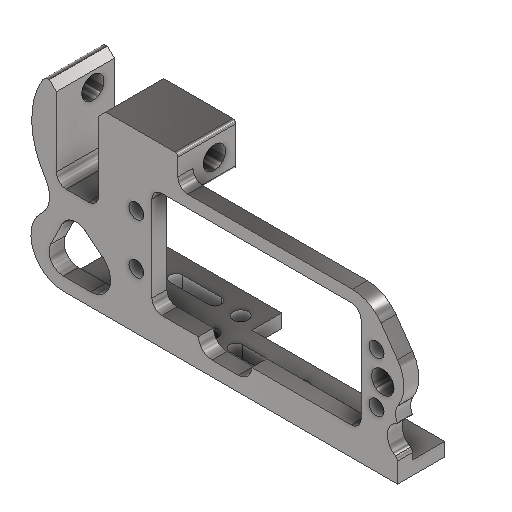
# Autodesk Inventor part: 650 서보모터 마운트
Saved by Autodesk Inventor 2026.2 (Build 302298010, 298A)
## iProperties
Created: 2026-03-24
Part Number: 650 서보모터 마운트
Material: 일반
Document SubType Name: Modeling
Designer: jh002
Density: 1 g/cm^3
Appearance: 기본값
Author: jh002
Autodesk Inventor part; units mm, degrees
ref_plane "YZ Plane" through (0, 0, 0) normal (1, 0, 0) x (0, 1, 0)
ref_plane "XZ Plane" through (0, 0, 0) normal (0, 1, 0) x (-1, 0, 0)
ref_plane "XY Plane" through (0, 0, 0) normal (0, 0, 1) x (1, 0, 0)
sketch "스케치1" plane through (0, 0, 0) normal (0, 1, 0) x (-1, 0, 0)
  line L0 (33.1, -7.725) -> (-33.1, -7.725)
  line L1 (-33.1, -7.725) -> (-33.1, 7.725)
  line L2 (-33.1, 7.725) -> (33.1, 7.725)
  line L3 (33.1, 7.725) -> (33.1, -7.725)
  line L4 (33.1, -7.725) -> (-33.1, 7.725) construction
  line L5 (-33.1, -7.725) -> (33.1, 7.725) construction
  line L6 (33.1, -1.675) -> (-33.1, -1.675)
  line L7 (5.4, -1.675) -> (5.4, -7.725)
  point P0 (0, 0)
  dimension "d0" = 66.2
  dimension "d1" = 15.45
  dimension "d2" = 9.4
  dimension "d3" = 38.5
  constraints: 16 end point, 4 point on line, 3 perpendicular, 2 midpoint, 2 parallel, 1 horizontal
  measures "d0" distance of L1.end L2.end
  measures "d1" distance of L0.end L1.end
  measures "d2" distance between parallel lines of L2 L6
  measures "d3" distance between parallel lines of L1 L7
extrude "돌출1" add sketch "스케치1" along normal blind 2.7 contours L0 L7 L6 L3 | L6 L1 L2 L3
sketch "스케치2" plane through (0, 0, 0) normal (0, -1, 0) x (1, 0, 0)
  line L0 (33.1, 7.725) -> (33.1, -1.675) projected
  line L1 (-33.1, 7.725) -> (33.1, 7.725) projected
  line L2 (-33.1, -7.725) -> (-33.1, 7.725) projected
  line L3 (-5.4, -7.725) -> (-33.1, -7.725) projected
  line L4 (-5.4, -1.675) -> (-5.4, -7.725) projected
  line L5 (33.1, -1.675) -> (-5.4, -1.675) projected
  circle A0 centre (27, 3.025) radius 1.5
  circle A1 centre (9, 3.025) radius 1.5
  circle A2 centre (-9, 3.025) radius 1.5
  line L6 (9, 3.025) -> (27, 3.025) construction
  line L7 (12.885, 3.025) -> (23.115, 3.025) construction
  line L8 (14.135, 4.275) -> (21.865, 4.275)
  line L9 (23.115, 3.025) -> (23.115, 3.025)
  line L10 (21.865, 1.775) -> (14.135, 1.775)
  line L11 (12.885, 3.025) -> (12.885, 3.025)
  line L12 (12.885, 4.275) -> (23.115, 1.775) construction
  line L13 (23.115, 4.275) -> (12.885, 1.775) construction
  arc A3 (14.135, 4.275) -> (12.885, 3.025) centre (14.135, 3.025) ccw
  arc A4 (12.885, 3.025) -> (14.135, 1.775) centre (14.135, 3.025) ccw
  arc A5 (21.865, 1.775) -> (23.115, 3.025) centre (21.865, 3.025) ccw
  arc A6 (23.115, 3.025) -> (21.865, 4.275) centre (21.865, 3.025) ccw
  line L14 (-9, 3.025) -> (9, 3.025) construction
  line L15 (-5.115, 3.025) -> (5.115, 3.025) construction
  line L16 (-3.865, 4.275) -> (3.865, 4.275)
  line L17 (5.115, 3.025) -> (5.115, 3.025)
  line L18 (3.865, 1.775) -> (-3.865, 1.775)
  line L19 (-5.115, 3.025) -> (-5.115, 3.025)
  line L20 (-5.115, 4.275) -> (5.115, 1.775) construction
  line L21 (5.115, 4.275) -> (-5.115, 1.775) construction
  arc A7 (-3.865, 4.275) -> (-5.115, 3.025) centre (-3.865, 3.025) ccw
  arc A8 (-5.115, 3.025) -> (-3.865, 1.775) centre (-3.865, 3.025) ccw
  arc A9 (3.865, 1.775) -> (5.115, 3.025) centre (3.865, 3.025) ccw
  arc A10 (5.115, 3.025) -> (3.865, 4.275) centre (3.865, 3.025) ccw
  line L22 (-23.115, 3.025) -> (-12.885, 3.025) construction
  line L23 (-21.865, 4.275) -> (-14.135, 4.275)
  line L24 (-14.135, 1.775) -> (-21.865, 1.775)
  line L25 (-23.115, 4.275) -> (-12.885, 1.775) construction
  line L26 (-12.885, 4.275) -> (-23.115, 1.775) construction
  arc A11 (-21.865, 4.275) -> (-23.115, 3.025) centre (-21.865, 3.025) ccw
  arc A12 (-23.115, 3.025) -> (-21.865, 1.775) centre (-21.865, 3.025) ccw
  arc A13 (-14.135, 1.775) -> (-12.885, 3.025) centre (-14.135, 3.025) ccw
  arc A14 (-12.885, 3.025) -> (-14.135, 4.275) centre (-14.135, 3.025) ccw
  line L27 (-9, 3.025) -> (-18, 3.025) construction
  circle A15 centre (-27, 3.025) radius 1.5
  line L28 (-7.8456, 0) -> (-28.9088, 0)
  circle A16 centre (-9, -3.025) radius 1.5
  arc A17 (-23.115, -3.025) -> (-21.865, -4.275) centre (-21.865, -3.025) ccw
  arc A18 (-21.865, -1.775) -> (-23.115, -3.025) centre (-21.865, -3.025) ccw
  line L29 (-21.865, -4.275) -> (-14.135, -4.275)
  line L30 (-14.135, -1.775) -> (-21.865, -1.775)
  line L31 (-23.115, -4.275) -> (-12.885, -1.775) construction
  line L32 (-12.885, -4.275) -> (-23.115, -1.775) construction
  arc A19 (-14.135, -4.275) -> (-12.885, -3.025) centre (-14.135, -3.025) ccw
  arc A20 (-12.885, -3.025) -> (-14.135, -1.775) centre (-14.135, -3.025) ccw
  line L33 (-23.115, -3.025) -> (-12.885, -3.025) construction
  line L34 (-9, -3.025) -> (-18, -3.025) construction
  circle A21 centre (-27, -3.025) radius 1.5
  point P0 (0, 0)
  point P1 (33.1, 3.025)
  point P2 (18, 3.025)
  point P3 (0, 3.025)
  point P4 (12.885, 3.025)
  point P5 (-5.115, 3.025)
  point P6 (-12.885, -3.025)
  point P7 (-12.885, 3.025)
  dimension "d6" = 3
  dimension "d7" = 6.1
  dimension "d8" = 3
  dimension "d9" = 18
  dimension "d10" = 3
  dimension "d11" = 18
  dimension "d24" = 10.23
  dimension "d25" = 1.25
  dimension "d26" = 10.23
  dimension "d27" = 1.25
  dimension "d135" = 10.23
  dimension "d136" = 1.25
  dimension "d137" = 9
  dimension "d138" = 3
  dimension "d139" = 18
  constraints: 58 end point, 32 point on circle, 27 point on line, 22 centre point, 21 symmetric about line, 20 tangent, 12 midpoint, 9 equal radius, 8 horizontal, 5 parallel, 2 perpendicular, 20 other
  measures "d6" diameter of A0
  measures "d7" distance of L6.end point (33.1, 3.025)
  measures "d8" diameter of A1
  measures "d9" distance of L6.end L6.start
  measures "d10" diameter of A2
  measures "d11" distance of L6.start L14.start
  measures "d24" distance of L7.start L7.end
  measures "d25" radius of A3
  measures "d26" distance of L15.start L15.end
  measures "d27" radius of A7
  measures "d135" distance of L22.start L22.end
  measures "d136" radius of A11
  measures "d137" distance of L14.start L27.end
  measures "d138" diameter of A15
  measures "d139" distance of A15.centre L14.start
sketch "스케치3" plane through (0, 2.7, 0) normal (0, 1, 0) x (1, 0, 0)
  line L0 (33.1, -7.725) -> (33.1, 1.675) projected
  line L1 (33.1, 1.675) -> (-5.4, 1.675) projected
  line L2 (-5.4, 1.675) -> (-5.4, 7.725) projected
  line L3 (-5.4, 7.725) -> (-33.1, 7.725) projected
  line L4 (-33.1, 7.725) -> (-33.1, -7.725) projected
  line L5 (-33.1, -7.725) -> (33.1, -7.725) projected
  line L6 (33.1, -4.725) -> (-33.1, -4.725)
  line L7 (-33.1, 7.725) -> (-33.1, -7.725) projected
  point P0 (0, 0)
  dimension "d19" = 3
  constraints: 2 end point, 2 point on line, 1 perpendicular
  measures "d19" distance between parallel lines of L5 L6
extrude "돌출2" add sketch "스케치3" along normal blind 40 contours L5 L4 L6 L0
extrude "돌출3" cut sketch "스케치2" against normal blind 10 contours A0 | A1 | A2 | L8 A6 A5 L10 A4 A3 | L16 A10 A9 L18 A8 A7 | L23 A14 A13 L24 A12 A11 | A15 | A16 | A18 L30 A20 A19 L29 A17 | A21
thread "스레드1" size "M2.5x0.45" class "6H" standard "ANSI Metric M Profile" full length
thread "스레드2" size "M2.5x0.45" class "6H" standard "ANSI Metric M Profile" full length
thread "스레드3" size "M2.5x0.45" class "6H" standard "ANSI Metric M Profile" full length
thread "스레드4" size "M2.5x0.45" class "6H" standard "ANSI Metric M Profile" full length
thread "스레드5" size "M2.5x0.45" class "6H" standard "ANSI Metric M Profile" full length
thread "스레드6" size "M2.5x0.45" class "6H" standard "ANSI Metric M Profile" full length
sketch "스케치4" plane through (-33.1, 0, 7.725) normal (0, 0, 1) x (1, 0, 0)
  line L0 (0, 0) -> (66.2, 0) projected
  line L1 (66.2, 0) -> (66.2, 42.7) projected
  line L2 (0, 42.7) -> (66.2, 42.7) projected
  line L3 (0, 0) -> (0, 42.7) projected
  line L4 (66.2, 4.5) -> (41.279, 4.5)
  arc A0 (66.2, 10.5) -> (66.2, 4.5) centre (67.3136, 7.5) ccw
  line L5 (66.2, 4.5) -> (66.2, 10.5)
  line L6 (66.2, 0) -> (66.2, 42.7) projected
  circle A1 centre (68.7981, 12) radius 3
  arc A2 (66.2, 13.513) -> (66.1805, 21.515) centre (60.4464, 17.5) ccw
  line L7 (0, 29.2) -> (66.2, 29.2)
  line L8 (60.7994, 29.2) -> (66.1805, 21.515)
  point P0 (33.1, 0)
  point P1 (66.2, 21.487)
  point P2 (66.2, 13.5)
  dimension "d48" = 6
  dimension "d44" = 4.5
  dimension "d45" = 6.4
  dimension "d47" = 6
  dimension "d50" = 7.5
  dimension "d51" = 14
  dimension "d52" = 13
  dimension "d53" = 29.2
  dimension "d54" = 125
  constraints: 8 end point, 7 point on line, 4 point on circle, 2 centre point, 2 perpendicular, 1 tangent, 4 other
  measures "d44" distance between parallel lines of L0 L4
  measures "d45" diameter of A0
  measures "d47" distance of L4.start L5.end
  measures "d50" distance from line of L4 point (68.798, 12)
  measures "d51" diameter of A2
  measures "d52" distance from line of L4 A2.centre
  measures "d53" distance between parallel lines of L0 L7
  measures "d54" angle of L8 L7
extrude "돌출4" cut sketch "스케치4" against normal blind 10 contours L3 L2 L1 L7 | A0 L1 | L7 L1 A2 L8 | A1 L1 picked at (66.115, 11.691)
extrude "돌출5" add sketch "스케치4" against normal blind 3 contours A2 L1
fillet "모깎기1" radius 7 1 edges at (27.6994, 29.2, 6.225)
sketch "스케치5" plane through (-33.1, 0, 7.725) normal (0, 0, 1) x (1, 0, 0)
  arc A0 (62.8895, 26.215) -> (57.1555, 29.2) centre (57.1555, 22.2) ccw projected
  line L0 (57.1555, 29.2) -> (0, 29.2) projected
  line L1 (0, 0) -> (0, 29.2) projected
  line L2 (0, 0) -> (66.2, 0) projected
  line L3 (66.2, 0) -> (66.2, 4.5) projected
  arc A1 (66.2, 10.5) -> (66.2, 4.5) centre (67.3136, 7.5) ccw projected
  arc A2 (66.2, 13.5) -> (66.2, 10.5) centre (68.7981, 12) ccw projected
  line L4 (66.2, 13.5) -> (66.2, 13.513) projected
  arc A3 (66.2, 13.513) -> (66.1805, 21.515) centre (60.4464, 17.5) ccw projected
  line L5 (66.1805, 21.515) -> (62.8895, 26.215) projected
  line L6 (56.0973, 0) -> (56.0973, 11.2)
  line L7 (66.2, 4.5) -> (62, 4.5)
  circle A4 centre (62, 11.2) radius 1.5
  circle A5 centre (62, 21.2) radius 1.5
  circle A6 centre (14, 11.2) radius 1.5
  circle A7 centre (14, 21.2) radius 1.5
  line L8 (17.09, 26.775) -> (58.91, 26.775)
  line L9 (58.91, 26.775) -> (58.91, 5.625)
  line L10 (17.09, 5.625) -> (17.09, 26.775)
  line L11 (17.09, 26.775) -> (58.91, 5.625) construction
  line L12 (58.91, 26.775) -> (17.09, 5.625) construction
  line L13 (26.41, 5.625) -> (26.41, 2.925)
  line L14 (26.41, 2.925) -> (37.05, 2.925)
  line L15 (36.965, 2.7) -> (29.235, 2.7) projected
  line L16 (37.05, 2.925) -> (37.05, 5.625)
  line L17 (58.91, 5.625) -> (37.05, 5.625)
  line L18 (26.41, 5.625) -> (17.09, 5.625)
  line L19 (62, 21.2) -> (62, 11.2)
  circle A8 centre (63.25, 16.2) radius 2.25
  point P0 (33.1, 0)
  point P1 (38, 16.2)
  dimension "d60" = 11.2
  dimension "d61" = 4.2
  dimension "d62" = 3
  dimension "d63" = 3
  dimension "d64" = 10
  dimension "d65" = 3
  dimension "d66" = 48
  dimension "d67" = 4.1805
  dimension "d68" = 4.2
  dimension "d69" = 3
  dimension "d70" = 21.15
  dimension "d71" = 41.82
  dimension "d72" = 2.7
  dimension "d73" = 9.32
  dimension "d74" = 10.64
  dimension "d76" = 4.5
  constraints: 26 end point, 6 perpendicular, 5 centre point, 4 parallel, 2 horizontal, 2 midpoint, 1 point on line, 1 other
  measures "d60" distance of L6.start L6.end
  measures "d61" distance of L3.end L7.end
  measures "d62" diameter of A4
  measures "d63" diameter of A5
  measures "d64" distance of L19.start L19.end
  measures "d65" diameter of A6
  measures "d66" distance of L19.end A6.centre
  measures "d67" horizontal distance of L5.start L19.start
  measures "d68" horizontal distance of A1.start L19.end
  measures "d69" diameter of A7
  measures "d70" distance of L10.start L8.start
  measures "d71" distance of L9.end L10.start
  measures "d72" distance of L13.start L13.end
  measures "d73" distance between parallel lines of L10 L13
  measures "d74" distance of L13.end L14.end
  measures "d76" diameter of A8
extrude "돌출6" cut sketch "스케치5" against normal blind 3 contours A4 | A5 | A6 | A7 | L8 L9 L17 L16 L14 L13 L18 L10 | A8 L19 | L19 A8
fillet "모깎기2" radius 2 4 edges at (-16.01, 26.775, 6.225) (25.81, 26.775, 6.225) (-16.01, 5.625, 6.225) (25.81, 5.625, 6.225)
fillet "모깎기3" radius 2.7 2 edges at (3.95, 2.925, 6.225) (-6.69, 2.925, 6.225)
fillet "모깎기4" radius 0.1 5 edges at (-5.4, 1.35, -7.725) (-33.1, 1.35, -7.725) (-19.25, 0, -7.725) (-19.25, 2.7, -7.725) (33.1, 10.5, 6.225)
fillet "모깎기5" radius 0.8 2 edges at (33.1, 4.5, 6.225) (33.1, 13.513, 6.225)
thread "스레드7" size "M2.5x0.45" class "6H" standard "ANSI Metric M Profile" full length
thread "스레드8" size "M2.5x0.45" class "6H" standard "ANSI Metric M Profile" full length
thread "스레드9" size "M2.5x0.45" class "6H" standard "ANSI Metric M Profile" full length
thread "스레드10" size "M2.5x0.45" class "6H" standard "ANSI Metric M Profile" full length
sketch "스케치6" plane through (33.1, 2.7, 4.725) normal (0, 0, -1) x (-1, 0, 0)
  line L0 (49.11, 22.075) -> (49.11, 4.925) projected
  line L1 (43.91, 24.075) -> (43.91, 32.525)
  line L2 (9.29, 24.075) -> (47.11, 24.075) projected
  line L3 (43.91, 32.525) -> (59.73, 32.525)
  line L4 (59.73, 32.525) -> (59.73, 15.225)
  line L5 (66.2, 26.5) -> (9.0445, 26.5) projected
  line L6 (59.73, 15.225) -> (68.18, 15.225)
  line L7 (68.18, 32.525) -> (70.48, 32.525)
  line L8 (43.91, 24.075) -> (56.91, 24.075)
  line L9 (56.91, 11.525) -> (69.5923, 11.525)
  line L10 (56.91, 24.075) -> (56.91, 11.525)
  arc A0 (49.11, 22.075) -> (47.11, 24.075) centre (47.11, 22.075) ccw projected
  line L11 (47.11, 24.075) -> (43.91, 24.075)
  line L12 (68.18, 32.525) -> (70.48, 32.525)
  arc A1 (70.3993, 15.1052) -> (70.48, 32.525) centre (57.5109, 23.875) ccw
  circle A2 centre (74.533, 12.2924) radius 5
  line L13 (43.91, 24.075) -> (56.91, 24.075)
  line L14 (68.18, 32.525) -> (68.18, 15.225)
  line L15 (56.91, 24.075) -> (59.73, 24.075)
  line L16 (59.73, 15.225) -> (59.73, 11.525)
  line L17 (68.18, 15.225) -> (68.18, 11.525)
  circle A3 centre (52.2, 8.5) radius 1.5 projected
  circle A4 centre (4.2, 8.5) radius 1.5 projected
  circle A5 centre (52.2, 18.5) radius 1.5 projected
  circle A6 centre (4.2, 18.5) radius 1.5 projected
  circle A7 centre (2.95, 13.5) radius 2.25 projected
  line L18 (49.11, 22.075) -> (49.11, 4.925) projected
  arc A8 (47.11, 2.925) -> (49.11, 4.925) centre (47.11, 4.925) ccw projected
  line L19 (47.11, 2.925) -> (39.79, 2.925) projected
  arc A9 (37.09, 0.225) -> (39.79, 2.925) centre (37.09, 2.925) ccw projected
  line L20 (37.09, 0.225) -> (31.85, 0.225) projected
  arc A10 (29.15, 2.925) -> (31.85, 0.225) centre (31.85, 2.925) ccw projected
  line L21 (29.15, 2.925) -> (9.29, 2.925) projected
  arc A11 (7.29, 4.925) -> (9.29, 2.925) centre (9.29, 4.925) ccw projected
  line L22 (7.29, 4.925) -> (7.29, 22.075) projected
  arc A12 (9.29, 24.075) -> (7.29, 22.075) centre (9.29, 22.075) ccw projected
  line L23 (9.29, 24.075) -> (47.11, 24.075) projected
  arc A13 (49.11, 22.075) -> (47.11, 24.075) centre (47.11, 22.075) ccw projected
  arc A14 (0.4173, 1.9899) -> (0, 1.2874) centre (0.8, 1.2874) ccw projected
  line L24 (0, 0) -> (0, 1.2874) projected
  line L25 (66.2, 0) -> (0, 0) projected
  line L26 (66.2, 0) -> (66.2, 26.5) projected
  line L27 (66.2, 26.5) -> (9.0445, 26.5) projected
  arc A15 (9.0445, 26.5) -> (3.3105, 23.515) centre (9.0445, 19.5) ccw projected
  line L28 (3.3105, 23.515) -> (0.0195, 18.815) projected
  arc A16 (0.0195, 18.815) -> (-0.052, 10.889) centre (5.7536, 14.8) ccw projected
  arc A17 (0, 10.8) -> (-0.052, 10.889) centre (-0.7154, 10.442) ccw projected
  arc A18 (0.0543, 7.8982) -> (0, 10.8) centre (-2.5981, 9.3) ccw projected
  arc A19 (0.0543, 7.8982) -> (0.1046, 7.7591) centre (0.1427, 7.8515) ccw projected
  arc A20 (0.4173, 1.9899) -> (0.1046, 7.7591) centre (-1.1136, 4.8) ccw projected
  point P0 (33.1, -2.7)
  point P1 (63.955, 15.225)
  point P2 (43.91, 26.5)
  point P3 (59.73, 26.5)
  point P4 (66.2, 15.225)
  dimension "d91" = 5.2
  dimension "d92" = 8.45
  dimension "d93" = 15.82
  dimension "d94" = 17.3
  dimension "d95" = 8.45
  dimension "d97" = 13
  dimension "d98" = 3.7
  dimension "d99" = 2.3
  dimension "d101" = 10
  constraints: 30 end point, 6 point on line, 4 point on circle, 4 vertical, 3 horizontal, 2 centre point, 2 collinear, 2 perpendicular, 1 midpoint, 1 tangent
  measures "d91" distance between parallel lines of L0 L1
  measures "d92" distance between parallel lines of L3 L2
  measures "d93" distance between parallel lines of L4 L1
  measures "d94" distance of L3.end L4.end
  measures "d95" distance of L4.end L6.end
  measures "d97" distance of L1.start L8.end
  measures "d98" distance from line of L9 point (63.955, 15.225)
  measures "d99" distance of L7.end L7.start
  measures "d101" diameter of A2
extrude "돌출7" add sketch "스케치6" along normal blind 8.6 and the other way blind 3 contours L2 L1 L5 L4 L15 L8 | L15 L4 L16 L9 L10 | L1 L3 L4 L5 | L16 L6 L26 L9 | L26 L6 L17 L9 | L17 L14 L7 A1 A2 L9
extrude "돌출8" cut sketch "스케치6" against normal blind 8.6 contours L4 L5 L26 L6
fillet "모깎기6" radius 0.6 2 edges at (-10.81, 35.225, 1.925) (-10.81, 26.775, 0.425)
fillet "모깎기7" radius 2 1 edges at (-10.81, 29.2, 6.225)
fillet "모깎기8" radius 5 1 edges at (-23.81, 26.775, 0.425)
fillet "모깎기9" radius 8 1 edges at (-23.81, 14.225, 0.425)
fillet "모깎기10" radius 0.5 1 edges at (-36.4923, 14.225, 1.925)
fillet "모깎기11" radius 1.5 1 edges at (-37.38, 35.225, 1.925)
chamfer "모따기1" distance 1.4 angle 45 2 edges at (-35.08, 35.225, 1.925) (-26.63, 35.225, 1.925)
sketch "스케치7" plane through (-10.81, 27.375, -3.875) normal (1, 0, 0) x (0, 0, -1)
  line L0 (0, 6.45) -> (-11.6, 6.45) projected
  line L1 (0, -9.45) -> (0, 6.45) projected
  line L2 (0, -9.45) -> (-11.6, -9.45) projected
  line L3 (-11.6, 6.45) -> (-11.6, -9.45) projected
  line L4 (0, 3.7557) -> (-4.3, 3.7557)
  line L5 (0, -0.6) -> (0, 0) projected
  line L6 (0, 0) -> (-8.6, 0) projected
  line L7 (-8.6, 0) -> (-8.6, -0.6) projected
  line L8 (-8.6, -0.6) -> (0, -0.6) projected
  line L9 (0, 7.85) -> (0, 6.45) projected
  line L10 (0, 6.45) -> (-11.6, 6.45) projected
  line L11 (-11.6, 6.45) -> (-11.6, 7.85) projected
  line L12 (-11.6, 7.85) -> (0, 7.85) projected
  line L13 (0, 7.85) -> (-11.6, 7.85) projected
  line L14 (-5.8, 7.85) -> (-5.8, 3.55)
  circle A0 centre (-4.3, 3.55) radius 2.25
  point P0 (-3.875, -27.375)
  dimension "d117" = 4.3
  dimension "d118" = 4.3
  dimension "d119" = 4.5
  constraints: 4 end point, 1 centre point, 1 midpoint, 1 perpendicular, 1 point on line, 1 vertical
  measures "d117" distance of L4.start L4.end
  measures "d118" distance of L14.start L14.end
  measures "d119" diameter of A0
extrude "돌출9" cut sketch "스케치7" against normal through all contours A0
sketch "스케치8" plane through (33.1, 2.7, 4.725) normal (0, 0, -1) x (-1, 0, 0)
  arc A0 (70.3993, 15.1052) -> (69.539, 12.0493) centre (74.533, 12.2924) ccw projected
  circle A1 centre (74.533, 12.2924) radius 5
  line L0 (47.11, 24.075) -> (9.29, 24.075) projected
  arc A2 (9.29, 24.075) -> (7.29, 22.075) centre (9.29, 22.075) ccw projected
  line L1 (7.29, 22.075) -> (7.29, 4.925) projected
  arc A3 (7.29, 4.925) -> (9.29, 2.925) centre (9.29, 4.925) ccw projected
  line L2 (9.29, 2.925) -> (29.15, 2.925) projected
  arc A4 (29.15, 2.925) -> (31.85, 0.225) centre (31.85, 2.925) ccw projected
  line L3 (31.85, 0.225) -> (37.09, 0.225) projected
  arc A5 (37.09, 0.225) -> (39.79, 2.925) centre (37.09, 2.925) ccw projected
  line L4 (39.79, 2.925) -> (47.11, 2.925) projected
  arc A6 (47.11, 2.925) -> (49.11, 4.925) centre (47.11, 4.925) ccw projected
  line L5 (49.11, 4.925) -> (49.11, 22.075) projected
  arc A7 (49.11, 22.075) -> (47.11, 24.075) centre (47.11, 22.075) ccw projected
  circle A8 centre (52.2, 8.5) radius 1.5 projected
  circle A9 centre (4.2, 8.5) radius 1.5 projected
  circle A10 centre (52.2, 18.5) radius 1.5 projected
  circle A11 centre (4.2, 18.5) radius 1.5 projected
  circle A12 centre (2.95, 13.5) radius 2.25 projected
  line L6 (59.73, 31.125) -> (58.33, 32.525) projected
  line L7 (59.73, 31.125) -> (59.73, 15.225) projected
  line L8 (59.73, 15.225) -> (68.18, 15.225) projected
  line L9 (68.18, 15.225) -> (68.18, 31.125) projected
  line L10 (69.58, 32.525) -> (68.18, 31.125) projected
  line L11 (69.58, 32.525) -> (69.6509, 32.525) projected
  arc A13 (70.9434, 31.7862) -> (69.6509, 32.525) centre (69.6509, 31.025) ccw projected
  arc A14 (70.3993, 15.1052) -> (70.9434, 31.7862) centre (57.5109, 23.875) ccw projected
  arc A15 (70.3993, 15.1052) -> (69.539, 12.0493) centre (74.533, 12.2924) ccw projected
  arc A16 (69.0396, 11.525) -> (69.539, 12.0493) centre (69.0396, 12.025) ccw projected
  line L12 (69.0396, 11.525) -> (66.2, 11.525) projected
  line L13 (66.2, -2.7) -> (66.2, 11.525) projected
  line L14 (66.2, -2.7) -> (0, -2.7) projected
  line L15 (0, -2.7) -> (0, 1.2874) projected
  arc A17 (0.4173, 1.9899) -> (0, 1.2874) centre (0.8, 1.2874) ccw projected
  arc A18 (0.4173, 1.9899) -> (0.1046, 7.7591) centre (-1.1136, 4.8) ccw projected
  arc A19 (0.0543, 7.8982) -> (0.1046, 7.7591) centre (0.1427, 7.8515) ccw projected
  arc A20 (0.0543, 7.8982) -> (0, 10.8) centre (-2.5981, 9.3) ccw projected
  arc A21 (0, 10.8) -> (-0.052, 10.889) centre (-0.7154, 10.442) ccw projected
  arc A22 (0.0195, 18.815) -> (-0.052, 10.889) centre (5.7536, 14.8) ccw projected
  line L16 (0.0195, 18.815) -> (3.3105, 23.515) projected
  arc A23 (9.0445, 26.5) -> (3.3105, 23.515) centre (9.0445, 19.5) ccw projected
  line L17 (9.0445, 26.5) -> (41.91, 26.5) projected
  arc A24 (41.91, 26.5) -> (43.91, 28.5) centre (41.91, 28.5) ccw projected
  line L18 (43.91, 28.5) -> (43.91, 31.925) projected
  arc A25 (44.51, 32.525) -> (43.91, 31.925) centre (44.51, 31.925) ccw projected
  line L19 (44.51, 32.525) -> (58.33, 32.525) projected
  arc A26 (66.7787, -2.7) -> (71.1616, 8.6) centre (66.7787, 3.8) ccw
  line L20 (66.2, -2.7) -> (66.7787, -2.7)
  point P0 (33.1, -2.7)
  dimension "d123" = 10
  dimension "d122" = 13
  constraints: 2 end point, 2 point on circle, 2 tangent, 1 centre point, 1 coincident, 4 other
  measures "d122" diameter of A26
extrude "돌출10" add sketch "스케치8" against normal blind 3 contours A1 A26 L20 L13 L12 A16
fillet "모깎기12" radius 2 2 edges at (-26.63, 17.925, 1.925) (-35.08, 17.925, 1.925)
sketch "스케치9" plane through (33.1, 2.7, 4.725) normal (0, 0, -1) x (-1, 0, 0)
  line L0 (38.6, -0.1) -> (66.1, -0.1) projected
  line L1 (64.9022, 11.525) -> (69.0396, 11.525) projected
  arc A0 (56.907, 19.2481) -> (64.9022, 11.525) centre (64.9022, 19.525) ccw projected
  arc A1 (66.7787, -2.7) -> (71.1616, 8.6) centre (66.7787, 3.8) ccw projected
  line L2 (66.7787, 3.8) -> (66.7787, 2.8)
  arc A2 (66.7787, -0.1) -> (69.3697, 4.1026) centre (66.7787, 2.8) ccw
  line L3 (53.116, 10.55) -> (79.6822, 10.55)
  line L4 (57.3287, -5.9451) -> (57.3287, 16.4375)
  arc A3 (66.959, 8.8975) -> (62.4009, 9.8896) centre (64.2787, 7.55) ccw
  arc A4 (58.8249, 7.0195) -> (61.3287, -0.1) centre (61.3287, 3.9) ccw
  line L5 (66.1, -0.1) -> (66.236, -0.1)
  line L6 (66.236, -0.1) -> (66.7787, -0.1)
  line L7 (58.8249, 7.0195) -> (62.4009, 9.8896)
  line L8 (66.959, 8.8975) -> (69.3697, 4.1026)
  point P0 (33.1, -2.7)
  dimension "d127" = 1
  dimension "d128" = 10.65
  dimension "d130" = 2.5
  constraints: 14 end point, 7 tangent, 6 point on circle, 3 centre point, 2 point on line, 2 vertical, 1 coincident, 1 horizontal, 1 other
  measures "d127" distance of L2.start L2.end
  measures "d128" distance between parallel lines of L0 L3
  measures "d130" distance from line of L2 A3.centre
extrude "돌출11" cut sketch "스케치9" against normal blind 3 contours A4 L7 A3 L8 A2 L6 L5 L0
